Autodesk Fusion 360 part; units mm, degrees
(part 3 of 3)
  spline S72 degree 3 poles (-35.684336, -13.811385) (-35.684331, -13.811388) (-35.684325, -13.811351) (-35.684299, -13.81133) (-35.684261, -13.811251) (-35.684206, -13.811162) (-35.684141, -13.811048) (-35.684054, -13.8109) (-35.683945, -13.810713) (-35.683771, -13.810416) (-35.683551, -13.810045) (-35.683286, -13.809602) (-35.68302, -13.80916) (-35.682662, -13.808573) (-35.682211, -13.807843) (-35.681663, -13.806972) (-35.680925, -13.805821) (-35.679986, -13.804398) (-35.678834, -13.802713) (-35.677656, -13.801054) (-35.676454, -13.799419) (-35.674822, -13.797277) (-35.672723, -13.794661) (-35.67011, -13.79162) (-35.667409, -13.788681) (-35.663701, -13.78491) (-35.65886, -13.780452) (-35.652739, -13.775519) (-35.646341, -13.77102) (-35.639692, -13.766959) (-35.632816, -13.763344) (-35.623389, -13.759132) (-35.611143, -13.755004) (-35.595938, -13.751945) (-35.580423, -13.750831) (-35.564791, -13.751724) (-35.543921, -13.755678) (-35.528879, -13.761857) (-35.519566, -13.767235) knots 0 0 0 0 0.00000162 0.00000648 0.00001296 0.00002591 0.00003886 0.00005181 0.00007769 0.00010357 0.00015528 0.00020695 0.00025856 0.00031013 0.00041314 0.00051596 0.0006186 0.00082337 0.00102748 0.00123094 0.0014338 0.00163607 0.00203895 0.00243979 0.00283878 0.0032361 0.00402622 0.00481145 0.00559278 0.00637109 0.00714714 0.00792156 0.00946707 0.01101258 0.01256227 0.01412112 0.01569566 0.01892218 0.01892218 0.01892218 0.01892218
  line L37 (-35.519566, -13.767235) -> (-33.563426, -14.896605)
  spline S73 degree 3 poles (-33.563426, -14.896605) (-33.563395, -14.896636) (-33.56331, -14.896666) (-33.563166, -14.896759) (-33.562902, -14.896907) (-33.562531, -14.897127) (-33.562086, -14.89739) (-33.561495, -14.897743) (-33.56076, -14.898188) (-33.559592, -14.89891) (-33.558148, -14.899828) (-33.556439, -14.900956) (-33.554754, -14.902109) (-33.552545, -14.903677) (-33.549845, -14.905697) (-33.546701, -14.90822) (-33.542656, -14.911697) (-33.537851, -14.916265) (-33.532493, -14.922086) (-33.52756, -14.928208) (-33.52306, -14.934606) (-33.517655, -14.943457) (-33.511998, -14.955107) (-33.507045, -14.969805) (-33.503986, -14.985013) (-33.502496, -15.005747) (-33.505725, -15.032207) (-33.513897, -15.052071) (-33.519276, -15.061385) knots 0 0 0 0 0.00001296 0.00002591 0.00005181 0.00010358 0.00015529 0.00020696 0.00031016 0.00041317 0.00061865 0.00082343 0.00102755 0.00123104 0.00163618 0.00203909 0.00243997 0.00323623 0.00402641 0.00481169 0.00559308 0.00637144 0.00792121 0.00946679 0.01101235 0.01256208 0.01568881 0.01891534 0.01891534 0.01891534 0.01891534
  line L38 (-33.519276, -15.061385) -> (-33.598646, -15.198865)
  spline S74 degree 3 poles (-33.598646, -15.198865) (-33.598676, -15.198895) (-33.598706, -15.19898) (-33.598799, -15.199125) (-33.598947, -15.199389) (-33.599168, -15.199759) (-33.59943, -15.200205) (-33.599784, -15.200796) (-33.600229, -15.201531) (-33.600951, -15.202698) (-33.601868, -15.204142) (-33.602996, -15.205852) (-33.604149, -15.207537) (-33.605717, -15.209746) (-33.607738, -15.212446) (-33.610261, -15.215589) (-33.613738, -15.219635) (-33.618306, -15.22444) (-33.624126, -15.229798) (-33.630248, -15.234731) (-33.636647, -15.239231) (-33.645498, -15.244636) (-33.657148, -15.250292) (-33.671846, -15.255245) (-33.687054, -15.258305) (-33.707787, -15.259795) (-33.734247, -15.256566) (-33.754112, -15.248393) (-33.763426, -15.243015) knots 0 0 0 0 0.00001296 0.00002591 0.00005181 0.00010358 0.00015529 0.00020696 0.00031016 0.00041317 0.00061865 0.00082343 0.00102755 0.00123104 0.00163618 0.00203909 0.00243997 0.00323623 0.00402641 0.00481169 0.00559308 0.00637144 0.00792121 0.00946679 0.01101235 0.01256208 0.01568881 0.01891534 0.01891534 0.01891534 0.01891534
  line L39 (-33.763426, -15.243015) -> (-35.719566, -14.113645)
  spline S75 degree 3 poles (-35.719566, -14.113645) (-35.719596, -14.113614) (-35.719681, -14.113584) (-35.719825, -14.113491) (-35.72009, -14.113343) (-35.72046, -14.113123) (-35.720906, -14.11286) (-35.721497, -14.112507) (-35.722232, -14.112062) (-35.723399, -14.11134) (-35.724843, -14.110422) (-35.726553, -14.109294) (-35.728237, -14.108141) (-35.730447, -14.106573) (-35.733146, -14.104553) (-35.73629, -14.10203) (-35.740335, -14.098553) (-35.745139, -14.093985) (-35.750498, -14.088164) (-35.75543, -14.082042) (-35.759929, -14.075644) (-35.765334, -14.066793) (-35.77099, -14.055143) (-35.775942, -14.040445) (-35.779001, -14.025237) (-35.780491, -14.004503) (-35.777263, -13.978044) (-35.769092, -13.958179) (-35.763716, -13.948865) knots 0 0 0 0 0.00001296 0.00002591 0.00005181 0.00010358 0.00015529 0.00020696 0.00031016 0.00041317 0.00061865 0.00082343 0.00102755 0.00123103 0.00163617 0.00203907 0.00243994 0.00323617 0.00402634 0.00481159 0.00559296 0.0063713 0.00792103 0.00946659 0.01101214 0.01256187 0.01568859 0.01891498 0.01891498 0.01891498 0.01891498
  line L40 (-15.768316, -25.493215) -> (-15.688936, -25.355735)
  spline S76 degree 3 poles (-15.688936, -25.355735) (-15.688936, -25.355746) (-15.688901, -25.355659) (-15.688869, -25.355628) (-15.688782, -25.355464) (-15.688677, -25.35529) (-15.688545, -25.355063) (-15.688371, -25.354766) (-15.688151, -25.354395) (-15.687798, -25.353804) (-15.687353, -25.353069) (-15.686811, -25.352193) (-15.686263, -25.351322) (-15.685525, -25.350171) (-15.684586, -25.348748) (-15.683434, -25.347063) (-15.681866, -25.344854) (-15.679846, -25.342154) (-15.677323, -25.339011) (-15.67471, -25.335969) (-15.672009, -25.333031) (-15.668301, -25.329259) (-15.66346, -25.324802) (-15.657339, -25.319869) (-15.650941, -25.315369) (-15.644292, -25.311309) (-15.637416, -25.307694) (-15.627989, -25.303482) (-15.615743, -25.299354) (-15.600538, -25.296295) (-15.585023, -25.295181) (-15.569391, -25.296074) (-15.548521, -25.300028) (-15.533479, -25.306207) (-15.524166, -25.311585) knots 0 0 0 0 0.00000324 0.00001296 0.00002591 0.00005181 0.00007769 0.00010357 0.00015528 0.00020695 0.00031013 0.00041314 0.00051596 0.0006186 0.00082337 0.00102748 0.00123094 0.00163605 0.00203893 0.00243978 0.00283877 0.00323608 0.00402621 0.00481143 0.00559277 0.00637108 0.00714712 0.00792155 0.00946706 0.01101257 0.01256226 0.01412111 0.01569564 0.01892216 0.01892216 0.01892216 0.01892216
  line L41 (-15.524166, -25.311585) -> (-13.568026, -26.440955)
  spline S77 degree 3 poles (-13.568026, -26.440955) (-13.567995, -26.440986) (-13.56791, -26.441016) (-13.567766, -26.441109) (-13.567502, -26.441257) (-13.567131, -26.441477) (-13.566686, -26.44174) (-13.566095, -26.442093) (-13.56536, -26.442538) (-13.564192, -26.44326) (-13.562748, -26.444178) (-13.561039, -26.445306) (-13.559354, -26.446459) (-13.557145, -26.448027) (-13.554445, -26.450047) (-13.551301, -26.45257) (-13.547256, -26.456047) (-13.542451, -26.460615) (-13.537093, -26.466436) (-13.53216, -26.472558) (-13.52766, -26.478956) (-13.522255, -26.487807) (-13.516598, -26.499457) (-13.511645, -26.514155) (-13.508586, -26.529363) (-13.507096, -26.550097) (-13.510325, -26.576557) (-13.518497, -26.596421) (-13.523876, -26.605735) knots 0 0 0 0 0.00001296 0.00002591 0.00005181 0.00010358 0.00015529 0.00020696 0.00031016 0.00041317 0.00061865 0.00082343 0.00102755 0.00123104 0.00163618 0.00203909 0.00243997 0.00323623 0.00402641 0.00481169 0.00559308 0.00637144 0.00792121 0.00946679 0.01101235 0.01256208 0.01568881 0.01891534 0.01891534 0.01891534 0.01891534
  line L42 (-13.523876, -26.605735) -> (-13.603246, -26.743215)
  spline S78 degree 3 poles (-13.603246, -26.743215) (-13.603276, -26.743245) (-13.603306, -26.74333) (-13.603399, -26.743475) (-13.603547, -26.743739) (-13.603768, -26.744109) (-13.60403, -26.744555) (-13.604384, -26.745146) (-13.604829, -26.745881) (-13.605551, -26.747048) (-13.606468, -26.748492) (-13.607596, -26.750202) (-13.608749, -26.751887) (-13.610317, -26.754096) (-13.612338, -26.756796) (-13.614861, -26.759939) (-13.618338, -26.763985) (-13.622906, -26.76879) (-13.628726, -26.774148) (-13.634848, -26.779081) (-13.641247, -26.783581) (-13.650098, -26.788986) (-13.661748, -26.794642) (-13.676446, -26.799595) (-13.691654, -26.802655) (-13.712387, -26.804145) (-13.738847, -26.800916) (-13.758712, -26.792743) (-13.768026, -26.787365) knots 0 0 0 0 0.00001296 0.00002591 0.00005181 0.00010358 0.00015529 0.00020696 0.00031016 0.00041317 0.00061865 0.00082343 0.00102755 0.00123104 0.00163618 0.00203909 0.00243997 0.00323623 0.00402641 0.00481169 0.00559308 0.00637144 0.00792121 0.00946679 0.01101235 0.01256208 0.01568881 0.01891534 0.01891534 0.01891534 0.01891534
  line L43 (-13.768026, -26.787365) -> (-15.724166, -25.657995)
  spline S79 degree 3 poles (-15.724166, -25.657995) (-15.724196, -25.657964) (-15.724281, -25.657934) (-15.724425, -25.657841) (-15.72469, -25.657693) (-15.72506, -25.657473) (-15.725506, -25.65721) (-15.726097, -25.656857) (-15.726832, -25.656412) (-15.727999, -25.65569) (-15.729443, -25.654772) (-15.731153, -25.653644) (-15.732837, -25.652491) (-15.735047, -25.650923) (-15.737746, -25.648903) (-15.74089, -25.64638) (-15.744935, -25.642903) (-15.749739, -25.638335) (-15.755098, -25.632514) (-15.76003, -25.626392) (-15.764529, -25.619994) (-15.769934, -25.611143) (-15.77559, -25.599493) (-15.780542, -25.584795) (-15.783601, -25.569587) (-15.785091, -25.548853) (-15.781863, -25.522394) (-15.773692, -25.502529) (-15.768316, -25.493215) knots 0 0 0 0 0.00001296 0.00002591 0.00005181 0.00010358 0.00015529 0.00020696 0.00031016 0.00041317 0.00061865 0.00082343 0.00102755 0.00123103 0.00163617 0.00203907 0.00243994 0.00323617 0.00402634 0.00481159 0.00559296 0.0063713 0.00792103 0.00946659 0.01101214 0.01256187 0.01568859 0.01891498 0.01891498 0.01891498 0.01891498
  line L44 (-31.109716, -9.236755) -> (-30.972226, -9.157375)
  spline S80 degree 3 poles (-30.972226, -9.157375) (-30.972184, -9.157364) (-30.972115, -9.157305) (-30.971963, -9.157227) (-30.971702, -9.157072) (-30.971327, -9.156861) (-30.970876, -9.156607) (-30.970275, -9.156272) (-30.969521, -9.155858) (-30.968313, -9.155208) (-30.966796, -9.154416) (-30.964965, -9.1535) (-30.963124, -9.152617) (-30.960662, -9.151488) (-30.957562, -9.15016) (-30.953806, -9.148699) (-30.948772, -9.146934) (-30.942414, -9.145058) (-30.934695, -9.143327) (-30.926927, -9.142116) (-30.919136, -9.141419) (-30.908769, -9.141163) (-30.895852, -9.142089) (-30.880648, -9.145148) (-30.865948, -9.150102) (-30.847248, -9.159178) (-30.825949, -9.175203) (-30.812832, -9.192211) (-30.807456, -9.201525) knots 0 0 0 0 0.00001296 0.00002591 0.00005181 0.00010357 0.00015528 0.00020695 0.00031013 0.00041314 0.0006186 0.00082337 0.00102748 0.00123095 0.00163606 0.00203895 0.0024398 0.003236 0.00402614 0.00481138 0.00559272 0.00637104 0.00792073 0.00946623 0.01101172 0.01256137 0.01568791 0.01891421 0.01891421 0.01891421 0.01891421
  line L45 (-30.807456, -9.201525) -> (-29.678076, -11.157665)
  spline S81 degree 3 poles (-29.678076, -11.157665) (-29.678071, -11.157662) (-29.678065, -11.157699) (-29.678039, -11.15772) (-29.678001, -11.157799) (-29.677946, -11.157888) (-29.677882, -11.158002) (-29.677796, -11.158151) (-29.677689, -11.158339) (-29.677519, -11.158639) (-29.677308, -11.159014) (-29.677056, -11.159466) (-29.676807, -11.159918) (-29.676477, -11.160521) (-29.67607, -11.161276) (-29.675591, -11.162186) (-29.674963, -11.163401) (-29.6742, -11.164926) (-29.673318, -11.166766) (-29.67247, -11.168616) (-29.671655, -11.170474) (-29.670616, -11.172959) (-29.6694, -11.176085) (-29.668073, -11.179869) (-29.66688, -11.183678) (-29.665467, -11.188774) (-29.664028, -11.195196) (-29.662817, -11.202963) (-29.662119, -11.210754) (-29.661864, -11.221122) (-29.66279, -11.234038) (-29.665849, -11.249243) (-29.670802, -11.263941) (-29.677595, -11.277934) (-29.686183, -11.291025) (-29.700041, -11.307122) (-29.712912, -11.317058) (-29.722226, -11.322435) knots 0 0 0 0 0.00000162 0.00000648 0.00001296 0.00002591 0.00003886 0.00005181 0.00007769 0.00010357 0.00015528 0.00020695 0.00025856 0.00031013 0.00041314 0.00051596 0.0006186 0.00082337 0.00102748 0.00123095 0.00143381 0.00163608 0.00203896 0.00243981 0.00283881 0.00323613 0.00402627 0.00481151 0.00559285 0.00637117 0.00792086 0.00946636 0.01101185 0.01256149 0.01412028 0.01569472 0.01892102 0.01892102 0.01892102 0.01892102
  line L46 (-29.722226, -11.322435) -> (-29.859716, -11.401815)
  spline S82 degree 3 poles (-29.859716, -11.401815) (-29.859757, -11.401826) (-29.859826, -11.401885) (-29.859979, -11.401963) (-29.860239, -11.402118) (-29.860615, -11.402329) (-29.861065, -11.402583) (-29.861667, -11.402919) (-29.86242, -11.403333) (-29.863628, -11.403983) (-29.865145, -11.404775) (-29.866976, -11.405692) (-29.868817, -11.406574) (-29.871279, -11.407704) (-29.874379, -11.409032) (-29.878136, -11.410493) (-29.883169, -11.412258) (-29.889527, -11.414136) (-29.897247, -11.415867) (-29.905014, -11.417078) (-29.912805, -11.417776) (-29.923172, -11.418031) (-29.936089, -11.417105) (-29.951293, -11.414046) (-29.965993, -11.409091) (-29.984693, -11.400014) (-30.005992, -11.383988) (-30.019109, -11.366979) (-30.024486, -11.357665) knots 0 0 0 0 0.00001296 0.00002591 0.00005181 0.00010358 0.00015529 0.00020696 0.00031016 0.00041317 0.00061864 0.00082343 0.00102754 0.00123102 0.00163616 0.00203905 0.00243992 0.00323614 0.00402629 0.00481153 0.00559287 0.0063712 0.00792089 0.0094664 0.01101191 0.01256159 0.01568823 0.01891458 0.01891458 0.01891458 0.01891458
  line L47 (-30.024486, -11.357665) -> (-31.153866, -9.401525)
  spline S83 degree 3 poles (-31.153866, -9.401525) (-31.153861, -9.401523) (-31.15389, -9.401498) (-31.153895, -9.401466) (-31.153945, -9.401393) (-31.153994, -9.401301) (-31.15406, -9.401188) (-31.154145, -9.401038) (-31.154252, -9.400851) (-31.154422, -9.400551) (-31.154634, -9.400176) (-31.154885, -9.399724) (-31.155135, -9.399272) (-31.155464, -9.398669) (-31.155871, -9.397914) (-31.15635, -9.397004) (-31.156978, -9.395789) (-31.157741, -9.394264) (-31.158623, -9.392424) (-31.159472, -9.390574) (-31.160286, -9.388716) (-31.161326, -9.386231) (-31.162541, -9.383105) (-31.163868, -9.379321) (-31.165062, -9.375512) (-31.166474, -9.370416) (-31.167914, -9.363994) (-31.169124, -9.356227) (-31.169822, -9.348436) (-31.170014, -9.340647) (-31.169706, -9.332885) (-31.168641, -9.322615) (-31.166092, -9.309946) (-31.161139, -9.295249) (-31.154347, -9.281256) (-31.145758, -9.268165) (-31.131901, -9.252068) (-31.11903, -9.242132) (-31.109716, -9.236755) knots 0 0 0 0 0.00000162 0.00000648 0.00001296 0.00002591 0.00003886 0.00005181 0.00007769 0.00010357 0.00015528 0.00020695 0.00025856 0.00031013 0.00041314 0.00051596 0.0006186 0.00082338 0.00102748 0.00123095 0.00143381 0.00163608 0.00203896 0.00243981 0.00283881 0.00323613 0.00402627 0.00481151 0.00559285 0.00637117 0.00714722 0.00792165 0.00946715 0.01101264 0.01256228 0.01412107 0.01569551 0.01892181 0.01892181 0.01892181 0.01892181
  line L48 (-19.565366, -29.232155) -> (-19.427876, -29.152775)
  spline S84 degree 3 poles (-19.427876, -29.152775) (-19.427834, -29.152764) (-19.427765, -29.152705) (-19.427613, -29.152627) (-19.427352, -29.152472) (-19.426977, -29.152261) (-19.426526, -29.152007) (-19.425925, -29.151672) (-19.425171, -29.151258) (-19.423963, -29.150608) (-19.422446, -29.149816) (-19.420615, -29.1489) (-19.418774, -29.148017) (-19.416312, -29.146888) (-19.413212, -29.14556) (-19.409456, -29.144099) (-19.404422, -29.142334) (-19.398064, -29.140458) (-19.390345, -29.138727) (-19.382577, -29.137516) (-19.374786, -29.136819) (-19.364419, -29.136563) (-19.351502, -29.137489) (-19.336298, -29.140548) (-19.321598, -29.145502) (-19.302898, -29.154578) (-19.281599, -29.170603) (-19.268482, -29.187611) (-19.263106, -29.196925) knots 0 0 0 0 0.00001296 0.00002591 0.00005181 0.00010357 0.00015528 0.00020695 0.00031013 0.00041314 0.0006186 0.00082337 0.00102748 0.00123095 0.00163606 0.00203895 0.0024398 0.003236 0.00402614 0.00481138 0.00559272 0.00637104 0.00792073 0.00946623 0.01101172 0.01256137 0.01568791 0.01891421 0.01891421 0.01891421 0.01891421
  line L49 (-19.263106, -29.196925) -> (-18.133726, -31.153065)
  spline S85 degree 3 poles (-18.133726, -31.153065) (-18.133726, -31.153054) (-18.133691, -31.153141) (-18.133659, -31.153172) (-18.133572, -31.153336) (-18.133468, -31.153511) (-18.133339, -31.15374) (-18.133169, -31.154039) (-18.132958, -31.154415) (-18.132622, -31.155016) (-18.132209, -31.155769) (-18.131558, -31.156977) (-18.130767, -31.158494) (-18.12985, -31.160326) (-18.128968, -31.162166) (-18.127838, -31.164629) (-18.126511, -31.167729) (-18.12505, -31.171485) (-18.123285, -31.176518) (-18.121408, -31.182877) (-18.119678, -31.190596) (-18.118467, -31.198364) (-18.117769, -31.206155) (-18.117514, -31.216522) (-18.11844, -31.229439) (-18.121499, -31.244644) (-18.126452, -31.259343) (-18.133245, -31.273337) (-18.141833, -31.286429) (-18.155691, -31.302528) (-18.168562, -31.312467) (-18.177876, -31.317845) knots 0 0 0 0 0.00000324 0.00001296 0.00002591 0.00005181 0.00007769 0.00010357 0.00015528 0.00020695 0.00031013 0.00041314 0.0006186 0.00082337 0.00102748 0.00123095 0.00163606 0.00203895 0.0024398 0.00323601 0.00402615 0.00481139 0.00559275 0.00637108 0.00792081 0.00946636 0.01101191 0.01256165 0.01412053 0.0156951 0.01892166 0.01892166 0.01892166 0.01892166
  line L50 (-18.177876, -31.317845) -> (-18.315366, -31.397215)
  spline S86 degree 3 poles (-18.315366, -31.397215) (-18.315407, -31.397226) (-18.315476, -31.397285) (-18.315629, -31.397363) (-18.315889, -31.397518) (-18.316265, -31.397729) (-18.316715, -31.397983) (-18.317317, -31.398319) (-18.31807, -31.398733) (-18.319278, -31.399383) (-18.320795, -31.400175) (-18.322626, -31.401092) (-18.324467, -31.401974) (-18.326929, -31.403104) (-18.330029, -31.404432) (-18.333786, -31.405893) (-18.338819, -31.407658) (-18.345177, -31.409536) (-18.352897, -31.411267) (-18.360664, -31.412478) (-18.368455, -31.413176) (-18.378822, -31.413431) (-18.391739, -31.412505) (-18.406943, -31.409446) (-18.421643, -31.404491) (-18.440343, -31.395414) (-18.461642, -31.379388) (-18.474759, -31.362379) (-18.480136, -31.353065) knots 0 0 0 0 0.00001296 0.00002591 0.00005181 0.00010358 0.00015529 0.00020696 0.00031016 0.00041317 0.00061864 0.00082343 0.00102754 0.00123102 0.00163616 0.00203905 0.00243992 0.00323614 0.00402629 0.00481153 0.00559287 0.0063712 0.00792089 0.0094664 0.01101191 0.01256159 0.01568823 0.01891458 0.01891458 0.01891458 0.01891458
  line L51 (-18.480136, -31.353065) -> (-19.609516, -29.396925)
  spline S87 degree 3 poles (-19.609516, -29.396925) (-19.609516, -29.396903) (-19.609553, -29.39687) (-19.609588, -29.396793) (-19.609668, -29.396664) (-19.609773, -29.396476) (-19.609902, -29.396251) (-19.610072, -29.395951) (-19.610284, -29.395576) (-19.610619, -29.394974) (-19.611033, -29.394221) (-19.611521, -29.393314) (-19.612, -29.392404) (-19.612628, -29.391189) (-19.613391, -29.389664) (-19.614273, -29.387824) (-19.615403, -29.385361) (-19.616731, -29.382261) (-19.618191, -29.378505) (-19.619518, -29.374721) (-19.620712, -29.370912) (-19.622124, -29.365816) (-19.623564, -29.359394) (-19.624774, -29.351627) (-19.625472, -29.343836) (-19.625727, -29.333468) (-19.624802, -29.320551) (-19.621742, -29.305347) (-19.616789, -29.290648) (-19.607713, -29.271948) (-19.591688, -29.250648) (-19.57468, -29.237532) (-19.565366, -29.232155) knots 0 0 0 0 0.00000648 0.00001296 0.00002591 0.00005181 0.00007769 0.00010357 0.00015528 0.00020695 0.00031013 0.00041314 0.00051596 0.0006186 0.00082337 0.00102748 0.00123095 0.00163606 0.00203895 0.0024398 0.0028388 0.00323612 0.00402625 0.00481149 0.00559283 0.00637116 0.00792085 0.00946635 0.01101183 0.01256148 0.01568803 0.01891432 0.01891432 0.01891432 0.01891432
  ellipse E4 centre (-24.526556, -20.368579) end of major axis (-24.526556, -20.753579) minor radius 0.385
  dimension "d26" = 0.6
extrude "Extrusão6" cut sketch "Esboço4" against normal blind 0.4 contours A1 | S0 picked at (-39.056267, -11.904387) picked at (-34.255783, -29.7978) bodies 2
extrude "Extrusão7" add sketch "Esboço4" against normal blind 0.4 contours A1 | S0 picked at (-39.056267, -11.904387) picked at (-34.255783, -29.7978) bodies 2
extrude "Extrusão8" add sketch "Esboço4" along normal blind 0.4 contours A1 | S0 picked at (-39.056267, -11.904387) picked at (-34.255783, -29.7978) bodies 2
copy_body "Copiar e colar corpos2" bodies 2 1 makes body 3 makes body 4
move_body "Mover3" bodies 3 4 to x (1, 0, 0) y (0, 1, 0) z (0, 0, 1) at (111, 2, 0)
move_body "Mover4" bodies 3 to x (1, 0, 0) y (0, 1, 0) z (0, 0, 1) at (-50.1, 0, 6.8)
fillet "Arredondamento2" radius 3 1 edges at (91, 39.885255, 0) on bodies 4
fillet "Arredondamento3" radius 3 1 edges at (80.4534, 39.798874, 0) on bodies 4
fillet "Arredondamento4" radius 3 1 edges at (80.4534, 4.201126, 0) on bodies 4
fillet "Arredondamento5" radius 3 1 edges at (91, 4.114745, 0) on bodies 4
scale "Escala1" [suppressed]
